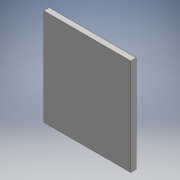
# Autodesk Inventor part: Hood_Top
Saved by Autodesk Inventor 2016 (Build 200138000, 138)
## iProperties
Created: 2018-09-18
Part Number: Hood_Top
Material: Generic
Document SubType Name: Modeling
Designer: Kyle
Density: 1 g/cm^3
Appearance: Default
Author: Kyle
Autodesk Inventor part; units mm, degrees
ref_plane "YZ Plane" through (0, 0, 0) normal (1, 0, 0) x (0, 1, 0)
ref_plane "XZ Plane" through (0, 0, 0) normal (0, 1, 0) x (-1, 0, 0)
ref_plane "XY Plane" through (0, 0, 0) normal (0, 0, 1) x (1, 0, 0)
sketch "Sketch1" plane through (0, 0, 0) normal (0, 1, 0) x (-1, 0, 0)
  line L0 (-36.5, -40) -> (-36.5, 40)
  line L1 (36.5, 40) -> (36.5, -40)
  line L2 (-36.5, 40) -> (36.5, -40) construction
  line L3 (36.5, 40) -> (-36.5, -40) construction
  line L4 (36.5, 40) -> (36.5, 13)
  line L5 (-36.5, 40) -> (36.5, 40)
  line L6 (-36.5, -40) -> (-9.5, -40)
  line L7 (-36.5, -40) -> (18.5, -40)
  line L8 (36.5, -40) -> (-36.5, -40)
  line L9 (31.9375, 35) -> (-31.5, 35)
  line L10 (-31.5, 35) -> (-31.5, -35)
  line L11 (31.5, 35) -> (31.5, -35)
  line L12 (31.5, -35) -> (-31.5, -35)
  dimension "d0" = 73
  dimension "d1" = 80
  dimension "d18" = 70
  dimension "d19" = 63
  constraints: 26 end point, 5 point on line, 2 parallel, 1 horizontal, 1 perpendicular
  measures "d0" distance of L1.end L0.start
  measures "d1" distance of L4.start L1.end
  measures "d18" distance of L11.start L11.end
  measures "d19" distance of L11.end L10.end
extrude "Extrusion1" add sketch "Sketch1" along normal blind 4 contours L11 L12 L10 L9
body "Solid1"
